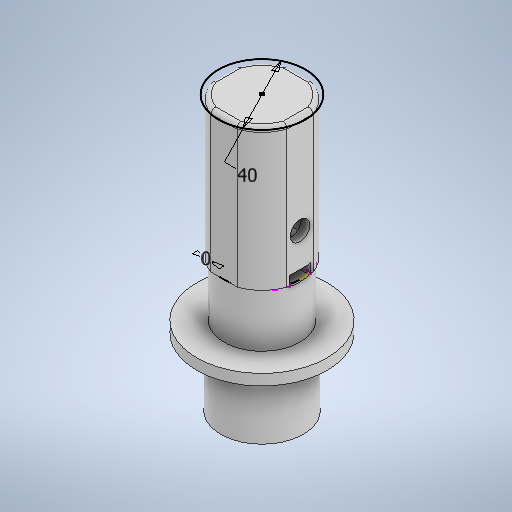
# Autodesk Inventor part: B2
Saved by Autodesk Inventor 2025 (Build 290162000, 162)
## iProperties
Created: 2025-01-09
Part Number: B2
Material: Générique
Document SubType Name: Modeling
Designer: adrie
Density: 1 g/cm^3
Appearance: Par défaut
Author: adrie
Autodesk Inventor part; units mm, degrees
ref_plane "YZ Plane" through (0, 0, 0) normal (1, 0, 0) x (0, 1, 0)
ref_plane "XZ Plane" through (0, 0, 0) normal (0, 1, 0) x (-1, 0, 0)
ref_plane "XY Plane" through (0, 0, 0) normal (0, 0, 1) x (1, 0, 0)
sketch "Esquisse1" plane through (0, 0, 0) normal (0, 1, 0) x (-1, 0, 0)
  circle A0 centre (0, 0) radius 19
  arc A1 (5.5841, 5.5882) -> (9.1184, 4.125) centre (9.1184, 9.125) ccw
  arc A2 (9.1184, -4.125) -> (5.5841, -5.5882) centre (9.1184, -9.125) ccw
  circle A3 centre (0, 0) radius 2.75
  arc A4 (5.5841, 5.5882) -> (5.5841, -5.5882) centre (0, 0) ccw
  circle A5 centre (9, 0) radius 1.5
  circle A6 centre (19.5, 0) radius 1.5
  line L0 (9.1184, 4.125) -> (25, 4.125)
  line L1 (9.1184, -4.125) -> (25, -4.125)
  circle A7 centre (23.5, 0) radius 1.5
  arc A8 (25, -4.125) -> (25, 4.125) centre (25, 0) ccw
  line L2 (0, 0) -> (39, 0) construction
  circle A9 centre (0, 0) radius 4.25
  dimension "d0" = 38
  dimension "d96" = 15.8
  dimension "d97" = 8.25
  dimension "d98" = 25
  dimension "d99" = 10
  dimension "d100" = 10
  dimension "d101" = 0
  dimension "d102" = 5.5
  dimension "d103" = 3
  dimension "d104" = 3
  dimension "d105" = 3
  dimension "d106" = 9
  dimension "d107" = 10.5
  dimension "d108" = 4
  dimension "d109" = 0
  dimension "d110" = 0
  dimension "d111" = 4.125
  dimension "d112" = 0
  dimension "d113" = 0
  dimension "d114" = 8.5
  constraints: 10 centre point, 8 point on circle, 6 end point, 4 tangent, 3 horizontal, 2 coincident, 2 point on line, 1 midpoint, 1 parallel, 1 other
  measures "d0" diameter of A0
  measures "d96" diameter of A4
  measures "d97" diameter of A8
  measures "d98" distance of point (0, 0) A8.centre
  measures "d99" diameter of A1
  measures "d100" diameter of A2
  measures "d101" distance from line of L2 A8.centre
  measures "d102" diameter of A3
  measures "d103" diameter of A5
  measures "d104" diameter of A6
  measures "d105" diameter of A7
  measures "d106" distance of point (0, 0) A5.centre
  measures "d107" distance of A5.centre A6.centre
  measures "d108" distance of A6.centre A7.centre
  measures "d109" distance of A9.centre L2.start
  measures "d110" distance of L2.start A9.centre
  measures "d111" distance from line of A7.centre L0
  measures "d112" distance of A0.centre point (0, 0)
  measures "d113" distance of point (0, 0) A0.centre
  measures "d114" diameter of A9
extrude "Extrusion1" add sketch "Esquisse1" along normal blind 9 contours L0 A1 A4 A2 L1 A0
sketch "Esquisse2" plane through (0, 9, 0) normal (0, 1, 0) x (1, 0, 0)
  circle A0 centre (0, 0) radius 19
  arc A1 (-18.5468, -4.125) -> (-18.5468, 4.125) centre (0, 0) ccw projected
  dimension "d116" = 0
  constraints: 1 centre point, 1 coincident
  measures "d116" radial gap between concentric circles of A1 A0
extrude "Extrusion2" add sketch "Esquisse2" along normal blind 22
sketch "Esquisse3" plane through (0, 31, 0) normal (0, 1, 0) x (1, 0, 0)
  circle A0 centre (0, 0) radius 19
  circle A1 centre (0, 0) radius 30
  circle A2 centre (0, 0) radius 19 projected
  dimension "d22" = 60
  dimension "d77" = 0
  constraints: 2 centre point, 2 coincident
  measures "d22" diameter of A1
  measures "d77" radial gap between concentric circles of A2 A0
extrude "Extrusion3" add sketch "Esquisse3" along normal blind 5 contours A0 | A1
sketch "Esquisse4" plane through (0, 36, 0) normal (0, 1, 0) x (1, 0, 0)
  circle A0 centre (0, 0) radius 17.5
  dimension "d25" = 35
  constraints: 1 centre point, 1 coincident
  measures "d25" diameter of A0
extrude "Extrusion4" add sketch "Esquisse4" along normal blind 25
sketch "Sketch6" plane through (0, 61, 0) normal (0, 1, 0) x (1, 0, 0)
  line L0 (-17.5, 17.5) -> (17.5, 17.5)
  line L1 (17.5, 17.5) -> (17.5, -17.5)
  line L2 (17.5, -17.5) -> (-17.5, -17.5)
  line L3 (-17.5, -17.5) -> (-17.5, 17.5)
  circle A0 centre (0, 0) radius 17.5 projected
  dimension "d33" = 35
  dimension "d34" = 35
  constraints: 8 end point, 2 parallel, 2 tangent, 1 horizontal, 1 perpendicular
  measures "d33" distance of L0.start L0.end
  measures "d34" distance of L0.end L1.end
extrude "Extrusion5" add sketch "Sketch6" along normal blind 65
sketch "Sketch7" plane through (-17.5, 61, -17.5) normal (-1, 0, 0) x (0, 0, 1)
  line L0 (7.35, 55) -> (27.65, 55)
  line L1 (27.65, 55) -> (27.65, 9)
  line L2 (27.65, 9) -> (7.35, 9)
  line L3 (7.35, 9) -> (7.35, 55)
  line L4 (0, 65) -> (35, 65) projected
  line L5 (35, 0) -> (35, 65) projected
  point P0 (17.5, -61)
  dimension "d39" = 20.3
  dimension "d40" = 46
  dimension "d41" = 10
  dimension "d42" = 7.35
  constraints: 8 end point, 2 parallel, 1 horizontal, 1 perpendicular
  measures "d39" distance of L0.start L0.end
  measures "d40" distance of L0.end L1.end
  measures "d41" distance between parallel lines of L4 L0
  measures "d42" distance between parallel lines of L5 L1
extrude "Extrusion6" cut sketch "Sketch7" against normal blind 31
sketch "Sketch8" plane through (13.5, 61, -17.5) normal (-1, 0, 0) x (0, 0, 1)
  circle A0 centre (17.5, 19.5) radius 4.5
  line L0 (27.65, 9) -> (7.35, 9) projected
  line L1 (27.65, 55) -> (27.65, 9) projected
  point P0 (17.5, -61)
  dimension "d45" = 9
  dimension "d46" = 10.5
  dimension "d47" = 10.15
  constraints: 1 centre point
  measures "d45" diameter of A0
  measures "d46" distance from line of L0 A0.centre
  measures "d47" distance from line of L1 A0.centre
extrude "Extrusion7" cut sketch "Sketch8" against normal blind 15
sketch "Sketch9" plane through (-17.5, 70, 10.15) normal (0, 1, 0) x (1, 0, 0)
  line L0 (29, 15.15) -> (19, 15.15)
  line L1 (19, 15.15) -> (19, 5.15)
  line L2 (19, 5.15) -> (29, 5.15)
  line L3 (29, 5.15) -> (29, 15.15)
  line L4 (0, 27.65) -> (0, -7.35) projected
  line L5 (0, 20.3) -> (31, 20.3) projected
  point P0 (17.5, 10.15)
  dimension "d50" = 10
  dimension "d51" = 10
  dimension "d52" = 19
  dimension "d53" = 5.15
  constraints: 8 end point, 2 parallel, 1 horizontal, 1 perpendicular
  measures "d50" distance of L2.end L0.start
  measures "d51" distance of L1.end L2.end
  measures "d52" distance between parallel lines of L4 L1
  measures "d53" distance between parallel lines of L0 L5
extrude "Extrusion8" cut sketch "Sketch9" against normal blind 10
sketch "Sketch10" plane through (11.5, 70, -5) normal (-1, 0, 0) x (0, 0, 1)
  line L0 (0, 0) -> (0, -10) projected
  line L1 (10, 0) -> (10, -10) projected
  line L2 (0, -10) -> (10, -10)
  line L3 (10, -10) -> (10, -5)
  line L4 (10, -5) -> (0, -5)
  line L5 (0, -5) -> (0, -10)
  point P0 (5, -70)
  point P1 (0, -5)
  constraints: 8 end point, 2 parallel, 1 horizontal, 1 midpoint, 1 perpendicular
extrude "Extrusion9" cut sketch "Sketch10" against normal blind 10
fillet "Fillet1" radius 10 2 edges at (-17.5, 93.5, 17.5) (-17.5, 93.5, -17.5)
sketch "Sketch11" plane through (-17.5, 116, -7.5) normal (-1, 0, 0) x (0, 0, 1)
  circle A0 centre (2.5, -49.4) radius 2.25
  circle A1 centre (12.5, -49.4) radius 2.25
  circle A2 centre (2.5, 0) radius 2.25
  circle A3 centre (12.5, 0) radius 2.25
  line L0 (0.0941, 0) -> (21.0941, 0)
  line L1 (17.65, 0) -> (17.65, -46) projected
  line L2 (15, -46) -> (0, -46) projected
  line L3 (0, 0) -> (15, 0) projected
  point P0 (7.5, -116)
  point P1 (10.25, 0)
  point P2 (14.75, 0)
  point P3 (0.25, 0)
  point P4 (4.75, 0)
  dimension "d61" = 4.5
  dimension "d62" = 10
  dimension "d63" = 10
  dimension "d68" = 0
  dimension "d69" = 0
  dimension "d70" = 5.15
  dimension "d71" = 3.4
  dimension "d72" = 3.4
  dimension "d73" = 0
  dimension "d74" = 5.15
  constraints: 4 centre point, 3 equal radius, 2 end point
  measures "d61" diameter of A3
  measures "d62" distance of A3.centre A2.centre
  measures "d63" distance of A1.centre A0.centre
  measures "d68" distance from line of L0 A2.centre
  measures "d69" distance from line of L0 A3.centre
  measures "d70" distance from line of L1 A1.centre
  measures "d71" distance from line of L2 A1.centre
  measures "d72" distance from line of L2 A0.centre
  measures "d73" distance between parallel lines of L3 L0
  measures "d74" distance from line of L1 A3.centre
extrude "Extrusion10" cut sketch "Sketch11" against normal blind 20 contours A0 | A1 | L0 A2 | A2 L0 | L0 A3 picked at (11.8141, 0.528)
sketch "Sketch12" plane through (0, 61, 0) normal (0, -1, 0) x (1, 0, 0)
  circle A0 centre (0, 0) radius 17.5
  arc A1 (0, -17.5) -> (17.5, 0) centre (0, 0) ccw projected
  point P0 (16.7705, -5)
  point P1 (16.7705, 5)
  point P2 (15, -9.0139)
  point P3 (15, 9.0139)
  dimension "d117" = 0
  constraints: 1 centre point, 1 coincident
  measures "d117" radial gap between concentric circles of A1 A0
chamfer "Chamfer2" distance 5 angle 45 1 edges at (11.5, 65, 0)
sketch "Sketch13" plane through (0, 61, 0) normal (0, -1, 0) x (1, 0, 0)
  circle A0 centre (0, 0) radius 40
  arc A1 (0, 17.5) -> (-17.5, 0) centre (0, 0) ccw projected
  arc A2 (-5.5841, -5.5882) -> (-5.5841, 5.5882) centre (0, 0) ccw projected
  circle A3 centre (0, 0) radius 18.5
  dimension "d124" = 80
  dimension "d130" = 1
  constraints: 2 centre point, 1 coincident
  measures "d124" diameter of A0
  measures "d130" radial gap between concentric circles of A1 A3
extrude "Extrusion11" cut sketch "Sketch13" against normal blind 80
fillet "Fillet5" radius 1 5 edges at (-7.2058, 0, 4.5053) (-13.8326, 0, 4.125) (-7.2058, 0, -4.5053) (-13.8326, 0, -4.125) (7.9, 0, 0)
fillet "Fillet6" radius 2 8 edges at (13.0815, 126, -13.0815) (17.5, 126, 0) (13.0815, 126, 13.0815) (0, 126, 17.5) (-13.0815, 126, 13.0815) (-17.5, 126, 0) (-13.0815, 126, -13.0815) (0, 126, -17.5)
sketch "Sketch14" plane through (0, 126, 0) normal (0, 1, 0) x (1, 0, 0)
  circle A0 centre (0, 0) radius 20
  dimension "d132" = 40
  constraints: 1 centre point, 1 coincident
  measures "d132" diameter of A0
equation "\"d100\" = d99"
equation "\"d72\" = d71"
